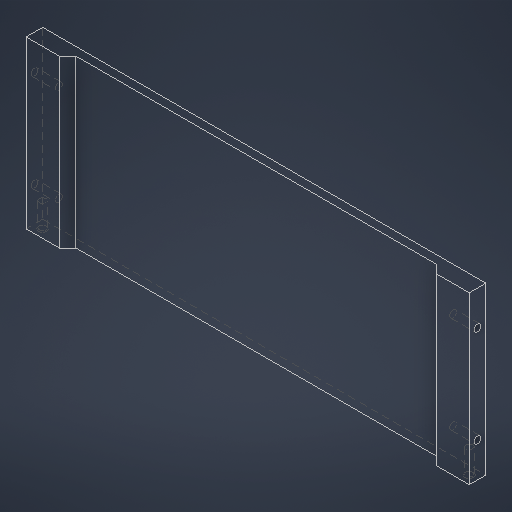
# Autodesk Inventor part: Prawa ściana
Saved by Autodesk Inventor 2026.1 (Build 301233020, 233B)
## iProperties
Created: 2026-02-25
Part Number: Prawa ściana
Material: Generic
Document SubType Name: Modeling
Designer: Jan
Density: 1 g/cm^3
Appearance: Default
Author: Jan
Autodesk Inventor part; units mm, degrees
ref_plane "YZ Plane" through (0, 0, 0) normal (1, 0, 0) x (0, 1, 0)
ref_plane "XZ Plane" through (0, 0, 0) normal (0, 1, 0) x (-1, 0, 0)
ref_plane "XY Plane" through (0, 0, 0) normal (0, 0, 1) x (1, 0, 0)
sketch "Sketch1" plane through (0, 0, 0) normal (0, 0, 1) x (1, 0, 0)
  line L0 (0, 0) -> (160, 0)
  line L1 (160, 0) -> (160, 60)
  line L2 (160, 60) -> (0, 60)
  line L3 (0, 60) -> (0, 0)
  dimension "d0" = 160
  dimension "d1" = 60
  constraints: 8 end point, 2 parallel, 1 horizontal, 1 perpendicular
  measures "d0" distance of L2.end L1.end
  measures "d1" distance of L1.end L0.end
extrude "Extrusion1" add sketch "Sketch1" along normal blind 6
sketch "Sketch2" plane through (0, 0, 0) normal (0, -1, 0) x (1, 0, 0)
  line L0 (3, 3) -> (157, 3) construction
  line L1 (160, 0) -> (0, 0) construction
  line L2 (0, 6) -> (160, 6) construction
  line L3 (160, 0) -> (160, 6) construction
  line L4 (0, 0) -> (0, 6) construction
  point P0 (0, 3)
  dimension "d4" = 3
  dimension "d5" = 6
  dimension "d6" = 3
  dimension "d7" = 3
  constraints: 2 end point, 1 midpoint, 1 parallel
  measures "d4" distance between parallel lines of L2 L0
  measures "d5" distance between parallel lines of L2 L1
  measures "d6" distance from line of L0.end L3
  measures "d7" distance of point (0, 3) L0.start
hole "Hole1" at (3, 0, 3) at (157, 0, 3) direction (0, 1, 0) diameter 2.459 depth 8.8 tip angle 118 thread size "M3x0.5" class "6H" standard "ISO Metric profile"
chamfer "Chamfer1" distance 0.3 angle 45 2 edges at (3, 0, 4.2295) (157, 0, 4.2295)
sketch "Sketch3" plane through (0, 60, 0) normal (0, 1, 0) x (1, 0, 0)
  line L0 (160, -6) -> (0, -6) projected
  line L1 (148, -6) -> (145, -3)
  line L2 (148, -6) -> (152.2426, -6) construction
  line L3 (145, -3) -> (15, -3)
  line L4 (160, 0) -> (0, 0) projected
  line L5 (15, -3) -> (12, -6)
  line L6 (12, -6) -> (148, -6)
  line L7 (160, 0) -> (160, -6) projected
  line L8 (0, 0) -> (0, -6) projected
  point P0 (12, -6)
  point P1 (0, -3)
  dimension "d18" = 135
  dimension "d19" = 3
  dimension "d22" = 15
  dimension "d23" = 130
  dimension "d24" = 15
  constraints: 10 end point, 2 parallel, 1 equal length, 1 horizontal, 1 midpoint, 1 perpendicular, 1 point on line
  measures "d18" angle of L2 L1
  measures "d19" distance between parallel lines of L3 L4
  measures "d22" distance from line of L7 L1.end
  measures "d23" distance of L1.end L3.end
  measures "d24" distance of point (0, -3) L3.end
extrude "Extrusion2" cut sketch "Sketch3" against normal through all contours L0 L5 L3 L1
sketch "Sketch6" plane through (160, 0, 0) normal (1, 0, 0) x (0, 0, -1)
  line L0 (-3, 60) -> (-3, 0) projected
  circle A0 centre (-3, 12.5) radius 1.5
  circle A1 centre (-3, 47.5) radius 1.5
  line L1 (0, 0) -> (-6, 0) projected
  line L2 (0, 60) -> (-6, 60) projected
  dimension "d34" = 3
  dimension "d35" = 3
  dimension "d36" = 35
  dimension "d37" = 12.5
  dimension "d38" = 60
  constraints: 2 centre point, 2 point on line
  measures "d34" diameter of A0
  measures "d35" diameter of A1
  measures "d36" distance of A1.centre A0.centre
  measures "d37" distance from line of L1 A0.centre
  measures "d38" distance between parallel lines of L2 L1
hole "Hole2" at (160, 12.5, 3) at (160, 47.5, 3) direction (-1, 0, 0) diameter 2.459 depth 8.8 tip angle 118 thread size "M3x0.5" class "6H" standard "ISO Metric profile"
sketch "Sketch7" plane through (0, 0, 0) normal (-1, 0, 0) x (0, 0, 1)
  line L0 (3, 60) -> (3, 0) projected
  circle A0 centre (3, 12.5) radius 1.5
  circle A1 centre (3, 47.5) radius 1.5
  line L1 (0, 60) -> (6, 60) projected
  line L2 (0, 0) -> (6, 0) projected
  dimension "d46" = 3
  dimension "d47" = 3
  dimension "d48" = 35
  dimension "d49" = 60
  dimension "d50" = 12.5
  constraints: 2 centre point, 2 point on line
  measures "d46" diameter of A0
  measures "d47" diameter of A1
  measures "d48" distance of A1.centre A0.centre
  measures "d49" distance between parallel lines of L1 L2
  measures "d50" distance from line of L2 A0.centre
hole "Hole3" at (0, 47.5, 3) at (0, 12.5, 3) direction (1, 0, 0) diameter 2.459 depth 8.8 tip angle 118 thread size "M3x0.5" class "6H" standard "ISO Metric profile"
equation "\"d4\" = 0.5 * d5"
equation "\"d7\" = d6"
equation "\"d22\" = d24"
equation "\"d37\" = -0.5 * d36 + 0.5 * d38"
equation "\"d50\" = -0.5 * d48 + 0.5 * d49"
body "Solid1"
